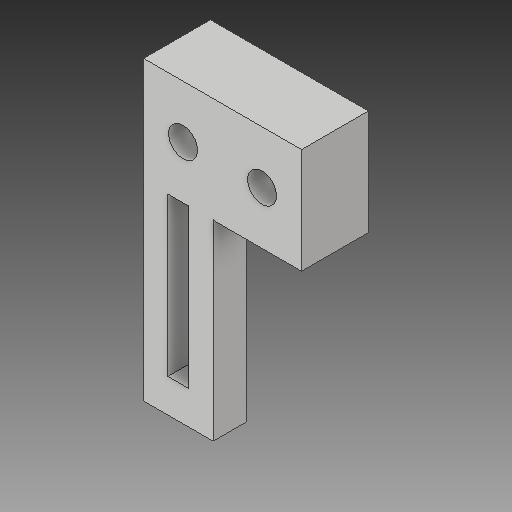
# Autodesk Inventor part: limitHolder
Saved by Autodesk Inventor 2019 (Build 230136000, 136)
## iProperties
Created: 2019-05-13
Part Number: limitHolder
Material: Generic
Document SubType Name: Modeling
Designer: Alex Jones
Density: 1 g/cm^3
Appearance: Default
Mass: 9.30322 g
Surface Area: 44.2751 cm^2
Volume: 9.30322 cm^3
Author: Alex Jones
Autodesk Inventor part; units mm, degrees
ref_plane "YZ Plane" through (0, 0, 0) normal (1, 0, 0) x (0, 1, 0)
ref_plane "XZ Plane" through (0, 0, 0) normal (0, 1, 0) x (-1, 0, 0)
ref_plane "XY Plane" through (0, 0, 0) normal (0, 0, 1) x (1, 0, 0)
sketch "Sketch1" plane through (0, 0, 0) normal (0, 0, 1) x (1, 0, 0)
  line L0 (0, 12.35) -> (250, 12.35) projected
  line L1 (0, 12.35) -> (0, 7.2) projected
  line L2 (0, 7.2) -> (250, 7.2) projected
  line L3 (250, 12.35) -> (250, 7.2) projected
  line L4 (250, 13.6) -> (0, 13.6) projected
  line L5 (0, -6.4) -> (250, -6.4) projected
  line L6 (250, -5.15) -> (0, -5.15) projected
  line L7 (250, 0) -> (250, -5.15) projected
  line L8 (0, 0) -> (250, 0) projected
  line L9 (0, 0) -> (0, -5.15) projected
  line L10 (250, -6.4) -> (220, -6.4)
  line L11 (220, -6.4) -> (220, 13.6)
  line L12 (220, 13.6) -> (250, 13.6)
  line L13 (250, 13.6) -> (250, -6.4)
  dimension "d0" = 30
  constraints: 8 end point, 2 parallel, 1 horizontal, 1 perpendicular, 1 point on line
  measures "d0" distance between parallel lines of L13 L11
extrude "Extrusion1" add sketch "Sketch1" along normal blind 6.35 contours L11 L4 L13 L0 | L0 L3 L2 L11 | L2 L13 L8 L11 | L8 L7 L6 L11 | L6 L13 L5 L11
sketch "Sketch2" plane through (0, 0, 6.35) normal (0, 0, 1) x (1, 0, 0)
  line L0 (250, 13.6) -> (220, 13.6) projected
  line L1 (220, -6.4) -> (250, -6.4) projected
  line L2 (220, 13.6) -> (250, -6.4)
  line L3 (235, 3.6) -> (250, 3.6)
  line L4 (250, -6.4) -> (250, 13.6) projected
  line L5 (235, 3.6) -> (220, 3.6)
  circle A0 centre (227.5, 3.6) radius 2.75
  circle A1 centre (242.5, 3.6) radius 2.75
  point P0 (0, 0)
  dimension "d3" = 5.5
  constraints: 6 end point, 4 midpoint, 2 centre point, 1 equal radius, 1 horizontal
  measures "d3" diameter of A1
extrude "Extrusion2" cut sketch "Sketch2" against normal blind 6.35 contours A0 L5 | L5 A0 | A1 L3 | L3 A1
sketch "Sketch3" plane through (0, 0, 6.35) normal (0, 0, 1) x (1, 0, 0)
  line L0 (220, -6.4) -> (220, 13.6) projected
  line L1 (220, -6.4) -> (224.604, -6.4)
  line L2 (224.604, -6.4) -> (224.604, -36.4)
  line L3 (224.604, -36.4) -> (220, -36.4)
  line L4 (220, -36.4) -> (220, -6.4)
  line L5 (250, -6.4) -> (220, -6.4) projected
  line L6 (233.2079, -6.4) -> (228.604, -6.4)
  line L7 (228.604, -6.4) -> (228.604, -36.4)
  line L8 (228.604, -36.4) -> (233.2079, -36.4)
  line L9 (233.2079, -36.4) -> (233.2079, -6.4)
  point P0 (0, 0)
  dimension "d6" = 30
  dimension "d7" = 4
  constraints: 16 end point, 4 parallel, 2 horizontal, 2 perpendicular, 2 point on line, 1 collinear
  measures "d6" distance of L8.end L6.start
  measures "d7" distance between parallel lines of L2 L7
extrude "Extrusion3" add sketch "Sketch3" against normal blind 6.35
sketch "Sketch4" plane through (0, 0, 6.35) normal (0, 0, 1) x (1, 0, 0)
  line L0 (233.2079, -6.4) -> (233.2079, -36.4) projected
  line L1 (233.2079, -36.4) -> (220, -36.4)
  line L2 (220, -36.4) -> (220, -42.75)
  line L3 (220, -42.75) -> (233.2079, -42.75)
  line L4 (233.2079, -42.75) -> (233.2079, -36.4)
  point P0 (0, 0)
  dimension "d10" = 6.35
  constraints: 8 end point, 2 parallel, 1 horizontal, 1 perpendicular
  measures "d10" distance of L3.end L0.end
extrude "Extrusion4" add sketch "Sketch4" against normal blind 6.35
sketch "Sketch5" plane through (0, 0, 0) normal (0, 0, -1) x (-1, 0, 0)
  line L0 (-228.604, -36.4) -> (-228.604, -6.4) projected
  line L1 (-228.604, -6.4) -> (-224.604, -6.4) projected
  line L2 (-224.604, -6.4) -> (-224.604, -36.4) projected
  line L3 (-224.604, -36.4) -> (-228.604, -36.4) projected
  circle A0 centre (-242.5, 3.6) radius 2.75 projected
  circle A1 centre (-227.5, 3.6) radius 2.75 projected
  line L4 (-233.2079, -6.4) -> (-233.2079, -42.75) projected
  line L5 (-233.2079, -42.75) -> (-220, -42.75) projected
  line L6 (-220, -42.75) -> (-220, 13.6) projected
  line L7 (-220, 13.6) -> (-250, 13.6) projected
  line L8 (-250, 13.6) -> (-250, -6.4) projected
  line L9 (-250, -6.4) -> (-233.2079, -6.4) projected
  line L10 (-233.2079, -6.4) -> (-233.2079, -42.75) projected
  line L11 (-233.2079, -6.4) -> (-220, -6.4)
  point P0 (0, 0)
  constraints: 2 end point, 1 horizontal, 1 point on line
extrude "Extrusion5" add sketch "Sketch5" along normal blind 6.35 contours L11 L9 L8 L7 L6 L1
body "Solid1"
